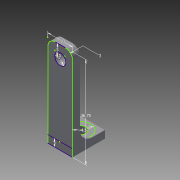
# Autodesk Inventor part: GearStand
Saved by Autodesk Inventor 2014 SP1 (Build 180222100, 222)
## iProperties
Created: 2014-06-07
Part Number: GearStand
Material: Generic
Document SubType Name: Modeling
Designer: Erin
Density: 1 g/cm^3
Appearance: Default
Author: Erin
Autodesk Inventor part; units mm, degrees
ref_plane "YZ Plane" through (0, 0, 0) normal (1, 0, 0) x (0, 1, 0)
ref_plane "XZ Plane" through (0, 0, 0) normal (0, 1, 0) x (-1, 0, 0)
ref_plane "XY Plane" through (0, 0, 0) normal (0, 0, 1) x (1, 0, 0)
sketch "Sketch1" plane through (0, 0, 0) normal (0, 1, 0) x (-1, 0, 0)
  circle A0 centre (0, 0) radius 2.25
  line L0 (-2, 5) -> (2, 5)
  line L1 (5, 2) -> (5, -31.75)
  line L2 (5, -31.75) -> (-5, -31.75)
  line L3 (-5, -31.75) -> (-5, 2)
  line L4 (-5, -28.75) -> (5, -28.75)
  arc A1 (-2, 5) -> (-5, 2) centre (-2, 2) ccw
  arc A2 (5, 2) -> (2, 5) centre (2, 2) ccw
  point P0 (-5, 5)
  point P1 (5, 5)
  dimension "d0" = 4.5
  dimension "d3" = 5
  dimension "d4" = 10
  dimension "d5" = 36.75
  dimension "d6" = 3
  dimension "d9" = 3
  constraints: 10 end point, 6 point on line, 4 point on circle, 4 tangent, 3 centre point, 2 parallel, 2 perpendicular, 1 coincident, 1 equal radius, 1 horizontal
  measures "d0" diameter of A0
  measures "d3" distance from line of A0.centre L0
  measures "d4" distance of point (-5, 5) point (5, 5)
  measures "d5" distance of L2.end point (-5, 5)
  measures "d6" distance between parallel lines of L2 L4
  measures "d9" radius of A1
extrude "Extrusion1" add sketch "Sketch1" along normal blind 3
extrude "Extrusion2" add sketch "Sketch1" along normal blind 13 contours L4 L1 L2 L3
sketch "Sketch2" plane through (-5, 3, -28.75) normal (0, 0, 1) x (1, 0, 0)
  circle A0 centre (5, 5) radius 2.25
  circle A1 centre (5, 5) radius 4.25
  point P0 (5, -3)
  dimension "d12" = 4.5
  dimension "d16" = 2
  constraints: 2 centre point, 1 coincident
  measures "d12" diameter of A0
  measures "d16" radial gap between concentric circles of A0 A1
extrude "Extrusion3" cut sketch "Sketch2" against normal blind 4 contours A0
fillet "Fillet1" radius 5 1 edges at (0, 3, -28.75)
extrude "Extrusion4" cut sketch "Sketch2" along normal blind 4
body "Solid1"
